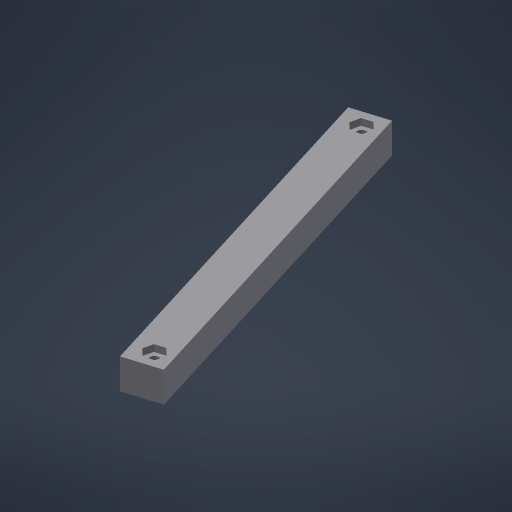
# Autodesk Inventor part: 3010 MOUNT PLATE RETAINER
Saved by Autodesk Inventor 2023.3 (Build 273359000, 359)
## iProperties
RuleStatus: InUse
AfterDocSave0: file://Part Number Cleaner
Created: 2021-11-16
Material: Generic
Catalog Web Link: https://www.janelia.org/
Vendor: HHMI: JRC - jET
Document SubType Name: Modeling
Designer: goulett
Density: 1 g/cm^3
Appearance: Default
Part Number: 3010 MOUNT PLATE RETAINER
LAB/DEPT: A. LEE (LAB)
DESIGN DEPARTMENT: HHMI: JRC - jET
ALTERED ITEM PART NUMBER: N/A
ALTERED ITEM VENDOR: N/A
ALTERED ITEM DESCRIPTION: N/A
Title: Standard
Author: goulett
Revision Number: 0
Autodesk Inventor part; units mm, degrees
ref_plane "YZ Plane" through (0, 0, 0) normal (1, 0, 0) x (0, 1, 0)
ref_plane "XZ Plane" through (0, 0, 0) normal (0, 1, 0) x (-1, 0, 0)
ref_plane "XY Plane" through (0, 0, 0) normal (0, 0, 1) x (1, 0, 0)
sketch "Sketch1" plane through (0, 0, 0) normal (0, 1, 0) x (-1, 0, 0)
  circle A0 centre (33.827, -45.1473) radius 1.143 projected
  circle A1 centre (11.7661, 26.4615) radius 1.143 projected
  line L0 (31.3076, -49.9102) -> (7.0032, 28.9809) projected
  line L1 (7.0032, 28.9809) -> (55.0834, 43.7932) projected
  line L2 (110.1987, -25.6058) -> (31.3076, -49.9102) projected
  line L3 (39.3181, -47.4424) -> (15.0137, 31.4487)
  line L4 (15.0137, 31.4487) -> (7.0032, 28.9809)
  line L5 (7.0032, 28.9809) -> (31.3076, -49.9102)
  point P0 (0, 0)
  point P1 (39.8036, -47.2928)
  point P2 (15.0137, 31.4487)
  dimension "d0" = 8.382
  constraints: 6 end point, 1 collinear, 1 parallel, 1 point on line
  measures "d0" distance between parallel lines of L0 L3
extrude "Extrusion1" add sketch "Sketch1" along normal blind 4.064
sketch "Sketch2" plane through (0, 0, 0) normal (0, -1, 0) x (1, 0, 0)
  line L0 (-13.8437, 22.9527) -> (-33.5699, -41.0776) projected
  line L1 (-16.4887, 27.953) -> (-13.8437, 22.9527) projected
  line L2 (-33.5699, -41.0776) -> (-38.5703, -43.7227) projected
  line L3 (-38.3328, -44.1717) -> (-33.1464, -41.4283)
  line L4 (-33.1464, -41.4283) -> (-13.2963, 23.0042)
  line L5 (-13.2963, 23.0042) -> (-16.0397, 28.1906)
  line L6 (-39.3181, -47.4424) -> (-15.0137, 31.4487) projected
  line L7 (-31.3076, -49.9102) -> (-39.3181, -47.4424) projected
  circle A0 centre (-11.7661, 26.4615) radius 1.143 projected
  circle A1 centre (-33.827, -45.1473) radius 1.143 projected
  line L8 (-7.0032, 28.9809) -> (-31.3076, -49.9102) projected
  line L9 (-15.0137, 31.4487) -> (-7.0032, 28.9809) projected
  point P0 (0, 0)
  point P1 (-37.7505, -43.8637)
  point P2 (-15.7317, 27.6083)
  point P3 (-16.0256, 28.164)
  point P4 (-38.3061, -44.1576)
  dimension "d3" = 0.508
  constraints: 6 end point, 2 other
  measures "d3" distance between parallel lines of L0 L4
extrude "Extrusion2" add sketch "Sketch2" along normal blind 3.175 contours L6 L9 L8 L7 L3 L4 L5
sketch "Sketch3" plane through (0, 4.064, 0) normal (0, 1, 0) x (1, 0, 0)
  circle A0 centre (-11.7661, -26.4615) radius 1.143 projected
  circle A1 centre (-33.827, 45.1473) radius 1.143 projected
  line L0 (-31.5846, 45.8381) -> (-32.1076, 43.5508)
  line L1 (-32.1076, 43.5508) -> (-34.3499, 42.86)
  line L2 (-34.3499, 42.86) -> (-36.0693, 44.4565)
  line L3 (-36.0693, 44.4565) -> (-35.5464, 46.7439)
  line L4 (-35.5464, 46.7439) -> (-33.3041, 47.4347)
  line L5 (-33.3041, 47.4347) -> (-31.5846, 45.8381)
  line L6 (-9.5237, -25.7707) -> (-10.0466, -28.058)
  line L7 (-10.0466, -28.058) -> (-12.289, -28.7488)
  line L8 (-12.289, -28.7488) -> (-14.0084, -27.1523)
  line L9 (-14.0084, -27.1523) -> (-13.4855, -24.8649)
  line L10 (-13.4855, -24.8649) -> (-11.2431, -24.1741)
  line L11 (-11.2431, -24.1741) -> (-9.5237, -25.7707)
  line L12 (-31.3076, 49.9102) -> (-39.3181, 47.4424) projected
  point P0 (0, 0)
  point P1 (-38.8933, 47.5732)
  dimension "d6" = 4.064
  dimension "d7" = 4.064
  constraints: 24 end point, 2 coincident, 2 parallel, 26 other
  measures "d6" distance between parallel lines of L7 L10
  measures "d7" distance from line of L3.end L1
extrude "Extrusion3" cut sketch "Sketch3" against normal blind 1.5875 contours A0 | L0 L1 L2 L3 L4 L5 | L6 L7 L8 L9 L10 L11
body "Solid1"
